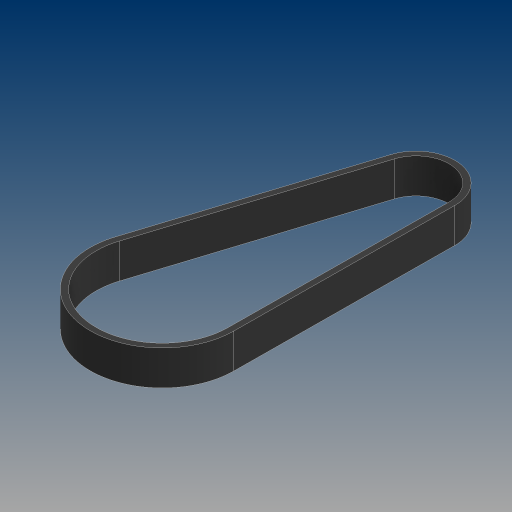
# Autodesk Inventor part: ELEV_028_BELT1
Saved by Autodesk Inventor 2024.3 (Build 283343000, 343)
## iProperties
Created: 2024-12-02
Part Number: ELEV_028_BELT1
Material: Rubber
Document SubType Name: Modeling
Designer: Kenji
Density: 0.93 g/cm^3
Appearance: Rubber - Black
Author: Kenji
Autodesk Inventor part; units mm, degrees
ref_plane "YZ Plane" through (0, 0, 0) normal (1, 0, 0) x (0, 1, 0)
ref_plane "XZ Plane" through (0, 0, 0) normal (0, 1, 0) x (-1, 0, 0)
ref_plane "XY Plane" through (0, 0, 0) normal (0, 0, 1) x (1, 0, 0)
sketch "Sketch1" plane through (0, 0, 0) normal (0, 1, 0) x (-1, 0, 0)
  circle A0 centre (0, 0) radius 14.3256 construction
  circle A1 centre (15.0854, 94.7166) radius 28.6512 construction
  line L0 (15.0854, 94.7166) -> (0, 0) construction
  line L1 (0, 0) -> (0, 94.7166) construction
  line L2 (0, 94.7166) -> (15.0854, 94.7166) construction
  line L3 (42.3895, 86.0345) -> (13.652, -4.3411)
  line L4 (-13.5648, 94.9463) -> (-14.3251, 0.1149)
  arc A2 (42.3895, 86.0345) -> (-13.5648, 94.9463) centre (15.0854, 94.7166) ccw
  arc A3 (-14.3251, 0.1149) -> (13.652, -4.3411) centre (0, 0) ccw
  arc A4 (-16.8651, 0.1352) -> (16.0726, -5.1107) centre (0, 0) ccw
  line L5 (16.0726, -5.1107) -> (44.8101, 85.2648)
  arc A5 (44.8101, 85.2648) -> (-16.1048, 94.9667) centre (15.0854, 94.7166) ccw
  line L6 (-16.1048, 94.9667) -> (-16.8651, 0.1352)
  point P0 (-16.8651, 0.1352)
  point P1 (-14.3251, 0.1149)
  dimension "d0" = 28.6512
  dimension "d1" = 57.3024
  dimension "d2" = 95.9104
  dimension "d3" = 94.7166
  dimension "d4" = 2.54
  constraints: 14 end point, 13 point on circle, 6 centre point, 6 tangent, 1 coincident, 1 concentric, 1 horizontal, 1 vertical, 3 other
  measures "d0" diameter of A0
  measures "d1" diameter of A1
  measures "d2" distance of L0.start L0.end
  measures "d3" distance of L0.end L1.end
  measures "d4" distance between parallel lines of L3 L5
extrude "Extrusion1" add sketch "Sketch1" along normal blind 15
equation "\"d1\" = 2 * d0"
body "Solid1"
